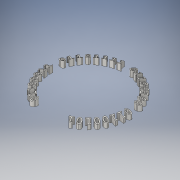
# Autodesk Inventor part: Team Pin Code-numbers
Saved by Autodesk Inventor 2016 (Build 200138000, 138)
## iProperties
Created: 2016-02-20
Part Number: Team Pin Code-numbers
Material: Generic
Document SubType Name: Modeling
Designer: RoksBot
Density: 1 g/cm^3
Appearance: White
Author: RoksBot
Autodesk Inventor part; units mm, degrees
ref_plane "YZ Plane" through (0, 0, 0) normal (1, 0, 0) x (0, 1, 0)
ref_plane "XZ Plane" through (0, 0, 0) normal (0, 1, 0) x (-1, 0, 0)
ref_plane "XY Plane" through (0, 0, 0) normal (0, 0, 1) x (1, 0, 0)
sketch "Sketch1" plane through (0, 0, 0) normal (0, 0, 1) x (1, 0, 0)
  line L0 (0, 0) -> (0, 8.6646) construction
  line L1 (20.9931, 1.27) -> (20.9931, 5.715)
  line L2 (20.9931, 5.715) -> (27.9781, 3.81)
  line L3 (27.9781, 3.81) -> (27.9781, 0)
  line L4 (27.9781, 0) -> (20.9931, 0)
  line L5 (20.9931, 1.27) -> (18.4531, 1.27)
  line L6 (18.4531, 1.27) -> (18.4531, 0)
  line L7 (18.4531, 0) -> (20.9931, 0)
  dimension "d0" = 20.9931
  dimension "d1" = 4.445
  dimension "d2" = 1.27
  dimension "d3" = 2.54
  dimension "d4" = 3.81
  dimension "d5" = 6.985
  constraints: 16 end point, 2 parallel, 2 perpendicular, 2 vertical, 1 horizontal, 1 horizontal alignment
  measures "d0" distance between parallel lines of L0 L1
  measures "d1" distance from line of L5 L1.end
  measures "d2" distance of L5.end L6.end
  measures "d3" distance between parallel lines of L1 L6
  measures "d4" distance of L2.end L3.end
  measures "d5" distance between parallel lines of L1 L3
revolve "Revolution1" add sketch "Sketch1" angle 360 about axis through (0, 0, 0) along (0, 1, 0)
sketch "Sketch2" plane through (0, 1.27, 0) normal (0, 1, 0) x (1, 0, 0)
  circle A0 centre (0, 0) radius 18.4531 projected
  circle A1 centre (0, 0) radius 27.9781 projected
  circle A2 centre (0, 0) radius 20.9931 projected
  circle A3 centre (0, 0) radius 22.8981
  line L0 (-12.5777, -21.7947) -> (-12.2792, -21.2089)
  spline S0 degree 2 poles (-12.2792, -21.2089) (-12.0125, -20.6853) (-10.9221, -20.0372) (-10.36, -20.3236) knots 0 0 0 1 2 2 2
  spline S1 degree 2 poles (-10.36, -20.3236) (-10.0346, -20.4894) (-9.7325, -21.001) (-9.7235, -21.9707) (-9.9421, -22.3997) knots 0 0 0 1 2 3 3 3
  line L1 (-9.9421, -22.3997) -> (-10.2405, -22.9854)
  spline S2 degree 2 poles (-10.2405, -22.9854) (-10.5058, -23.5061) (-11.5947, -24.1587) (-12.1568, -23.8723) knots 0 0 0 1 2 2 2
  spline S3 degree 2 poles (-12.1568, -23.8723) (-12.4793, -23.708) (-12.7828, -23.1994) (-12.7977, -22.2266) (-12.5777, -21.7947) knots 0 0 0 1 2 3 3 3
  spline S4 degree 2 poles (-12.0422, -22.0675) (-12.2653, -22.5054) (-12.1885, -22.9544) knots 0 0 0 1 1 1
  spline S5 degree 2 poles (-12.1885, -22.9544) (-12.1414, -23.2057) (-11.8899, -23.3338) knots 0 0 0 1 1 1
  spline S6 degree 2 poles (-11.8899, -23.3338) (-11.6444, -23.4589) (-11.3895, -23.3391) knots 0 0 0 1 1 1
  spline S7 degree 2 poles (-11.3895, -23.3391) (-11.0021, -23.1564) (-10.776, -22.7126) knots 0 0 0 1 1 1
  line L2 (-10.776, -22.7126) -> (-10.4776, -22.1268)
  spline S8 degree 2 poles (-10.4776, -22.1268) (-10.253, -21.686) (-10.3342, -21.2385) knots 0 0 0 1 1 1
  spline S9 degree 2 poles (-10.3342, -21.2385) (-10.3784, -20.9887) (-10.6328, -20.859) knots 0 0 0 1 1 1
  spline S10 degree 2 poles (-10.6328, -20.859) (-10.8754, -20.7355) (-11.1302, -20.8553) knots 0 0 0 1 1 1
  spline S11 degree 2 poles (-11.1302, -20.8553) (-11.5177, -21.038) (-11.7438, -21.4817) knots 0 0 0 1 1 1
  line L3 (-11.7438, -21.4817) -> (-12.0422, -22.0675)
  line L4 (-15.9925, -21.4944) -> (-14.0587, -18.8322)
  line L5 (-14.0587, -18.8322) -> (-14.5503, -18.4751)
  spline S12 degree 2 poles (-14.5503, -18.4751) (-14.733, -18.3425) (-14.7859, -18.0989) (-14.7059, -17.9887) knots 0 0 0 1 2 2 2
  spline S13 degree 2 poles (-14.7059, -17.9887) (-14.6259, -17.8786) (-14.3798, -17.8562) (-14.1971, -17.9889) knots 0 0 0 1 2 2 2
  line L6 (-14.1971, -17.9889) -> (-12.7277, -19.0563)
  spline S14 degree 2 poles (-12.7277, -19.0563) (-12.545, -19.189) (-12.4922, -19.4325) (-12.5722, -19.5427) knots 0 0 0 1 2 2 2
  spline S15 degree 2 poles (-12.5722, -19.5427) (-12.6522, -19.6528) (-12.8982, -19.6752) (-13.0809, -19.5425) knots 0 0 0 1 2 2 2
  line L7 (-13.0809, -19.5425) -> (-13.5725, -19.1854)
  line L8 (-13.5725, -19.1854) -> (-15.0457, -21.2136)
  line L9 (-15.0457, -21.2136) -> (-14.5286, -21.4169)
  spline S16 degree 2 poles (-14.5286, -21.4169) (-14.4023, -21.4635) (-14.3513, -21.5005) knots 0 0 0 1 1 1
  spline S17 degree 2 poles (-14.3513, -21.5005) (-14.2573, -21.5688) (-14.2303, -21.8141) (-14.3083, -21.9216) knots 0 0 0 1 2 2 2
  spline S18 degree 2 poles (-14.3083, -21.9216) (-14.3786, -22.0183) (-14.558, -22.0562) (-14.7477, -21.9841) knots 0 0 0 1 2 2 2
  line L10 (-14.7477, -21.9841) -> (-15.9925, -21.4944)
  line L11 (-19.1566, -18.7295) -> (-16.8304, -16.4024)
  line L12 (-16.8304, -16.4024) -> (-17.2601, -15.9728)
  spline S19 degree 2 poles (-17.2601, -15.9728) (-17.4198, -15.8132) (-17.4339, -15.5643) (-17.3377, -15.4681) knots 0 0 0 1 2 2 2
  spline S20 degree 2 poles (-17.3377, -15.4681) (-17.2415, -15.3718) (-16.9949, -15.3882) (-16.8353, -15.5478) knots 0 0 0 1 2 2 2
  line L13 (-16.8353, -15.5478) -> (-15.5508, -16.8318)
  spline S21 degree 2 poles (-15.5508, -16.8318) (-15.3911, -16.9914) (-15.377, -17.2403) (-15.4732, -17.3365) knots 0 0 0 1 2 2 2
  spline S22 degree 2 poles (-15.4732, -17.3365) (-15.5694, -17.4328) (-15.816, -17.4164) (-15.9756, -17.2568) knots 0 0 0 1 2 2 2
  line L14 (-15.9756, -17.2568) -> (-16.4054, -16.8273)
  line L15 (-16.4054, -16.8273) -> (-18.1776, -18.6002)
  line L16 (-18.1776, -18.6002) -> (-17.6986, -18.8818)
  spline S23 degree 2 poles (-17.6986, -18.8818) (-17.5812, -18.9475) (-17.5366, -18.9921) knots 0 0 0 1 1 1
  spline S24 degree 2 poles (-17.5366, -18.9921) (-17.4544, -19.0743) (-17.4661, -19.3208) (-17.56, -19.4147) knots 0 0 0 1 2 2 2
  spline S25 degree 2 poles (-17.56, -19.4147) (-17.6445, -19.4993) (-17.8276, -19.5087) (-18.0037, -19.4078) knots 0 0 0 1 2 2 2
  line L17 (-18.0037, -19.4078) -> (-19.1566, -18.7295)
  line L18 (-21.0982, -13.7139) -> (-20.5665, -13.3273)
  spline S26 degree 2 poles (-20.5665, -13.3273) (-20.0911, -12.9818) (-18.8254, -12.899) (-18.4545, -13.4093) knots 0 0 0 1 2 2 2
  spline S27 degree 2 poles (-18.4545, -13.4093) (-18.2397, -13.7047) (-18.2027, -14.2977) (-18.6347, -15.1659) (-19.0242, -15.449) knots 0 0 0 1 2 3 3 3
  line L19 (-19.0242, -15.449) -> (-19.5559, -15.8355)
  spline S28 degree 2 poles (-19.5559, -15.8355) (-20.0286, -16.1792) (-21.295, -16.2665) (-21.666, -15.7562) knots 0 0 0 1 2 2 2
  spline S29 degree 2 poles (-21.666, -15.7562) (-21.8788, -15.4635) (-21.9185, -14.8725) (-21.4903, -13.9989) (-21.0982, -13.7139) knots 0 0 0 1 2 3 3 3
  spline S30 degree 2 poles (-20.7449, -14.2) (-21.1423, -14.4889) (-21.2777, -14.9239) knots 0 0 0 1 1 1
  spline S31 degree 2 poles (-21.2777, -14.9239) (-21.3497, -15.1692) (-21.1838, -15.3975) knots 0 0 0 1 1 1
  spline S32 degree 2 poles (-21.1838, -15.3975) (-21.0218, -15.6204) (-20.7403, -15.6293) knots 0 0 0 1 1 1
  spline S33 degree 2 poles (-20.7403, -15.6293) (-20.3121, -15.6423) (-19.9093, -15.3494) knots 0 0 0 1 1 1
  line L20 (-19.9093, -15.3494) -> (-19.3775, -14.9629)
  spline S34 degree 2 poles (-19.3775, -14.9629) (-18.9774, -14.672) (-18.8467, -14.2363) knots 0 0 0 1 1 1
  spline S35 degree 2 poles (-18.8467, -14.2363) (-18.7727, -13.9936) (-18.9406, -13.7627) knots 0 0 0 1 1 1
  spline S36 degree 2 poles (-18.9406, -13.7627) (-19.1007, -13.5425) (-19.3821, -13.5336) knots 0 0 0 1 1 1
  spline S37 degree 2 poles (-19.3821, -13.5336) (-19.8103, -13.5206) (-20.2131, -13.8134) knots 0 0 0 1 1 1
  line L21 (-20.2131, -13.8134) -> (-20.7449, -14.2)
  line L22 (-22.983, -10.2463) -> (-22.3974, -9.9477)
  spline S38 degree 2 poles (-22.3974, -9.9477) (-21.8738, -9.6807) (-20.6107, -9.7969) (-20.3241, -10.3589) knots 0 0 0 1 2 2 2
  spline S39 degree 2 poles (-20.3241, -10.3589) (-20.1582, -10.6842) (-20.2144, -11.2757) (-20.7769, -12.0656) (-21.2058, -12.2844) knots 0 0 0 1 2 3 3 3
  line L23 (-21.2058, -12.2844) -> (-21.7914, -12.583)
  spline S40 degree 2 poles (-21.7914, -12.583) (-22.312, -12.8485) (-23.5765, -12.7368) (-23.8631, -12.1748) knots 0 0 0 1 2 2 2
  spline S41 degree 2 poles (-23.8631, -12.1748) (-24.0276, -11.8524) (-23.9743, -11.2624) (-23.4149, -10.4665) (-22.983, -10.2463) knots 0 0 0 1 2 3 3 3
  spline S42 degree 2 poles (-22.71, -10.7817) (-23.1478, -11.0049) (-23.3495, -11.4134) knots 0 0 0 1 1 1
  spline S43 degree 2 poles (-23.3495, -11.4134) (-23.459, -11.6444) (-23.3308, -11.8958) knots 0 0 0 1 1 1
  spline S44 degree 2 poles (-23.3308, -11.8958) (-23.2056, -12.1413) (-22.929, -12.1941) knots 0 0 0 1 1 1
  spline S45 degree 2 poles (-22.929, -12.1941) (-22.5081, -12.2739) (-22.0644, -12.0476) knots 0 0 0 1 1 1
  line L24 (-22.0644, -12.0476) -> (-21.4788, -11.749)
  spline S46 degree 2 poles (-21.4788, -11.749) (-21.0381, -11.5242) (-20.8408, -11.1143) knots 0 0 0 1 1 1
  spline S47 degree 2 poles (-20.8408, -11.1143) (-20.7298, -10.8863) (-20.8595, -10.6319) knots 0 0 0 1 1 1
  spline S48 degree 2 poles (-20.8595, -10.6319) (-20.9832, -10.3893) (-21.2598, -10.3366) knots 0 0 0 1 1 1
  spline S49 degree 2 poles (-21.2598, -10.3366) (-21.6807, -10.2568) (-22.1244, -10.483) knots 0 0 0 1 1 1
  line L25 (-22.1244, -10.483) -> (-22.71, -10.7817)
  line L26 (-24.3025, -6.5267) -> (-23.6773, -6.3233)
  spline S50 degree 2 poles (-23.6773, -6.3233) (-23.1185, -6.1414) (-21.8891, -6.4537) (-21.6939, -7.0536) knots 0 0 0 1 2 2 2
  spline S51 degree 2 poles (-21.6939, -7.0536) (-21.5809, -7.4009) (-21.7288, -7.9763) (-22.4079, -8.6686) (-22.8657, -8.8176) knots 0 0 0 1 2 3 3 3
  line L27 (-22.8657, -8.8176) -> (-23.4909, -9.021)
  spline S52 degree 2 poles (-23.4909, -9.021) (-24.0465, -9.2018) (-25.2781, -8.8937) (-25.4733, -8.2938) knots 0 0 0 1 2 2 2
  spline S53 degree 2 poles (-25.4733, -8.2938) (-25.5852, -7.9497) (-25.4404, -7.3753) (-24.7634, -6.6767) (-24.3025, -6.5267) knots 0 0 0 1 2 3 3 3
  spline S54 degree 2 poles (-24.1165, -7.0982) (-24.5838, -7.2502) (-24.8469, -7.6221) knots 0 0 0 1 1 1
  spline S55 degree 2 poles (-24.8469, -7.6221) (-24.9912, -7.8332) (-24.9038, -8.1015) knots 0 0 0 1 1 1
  spline S56 degree 2 poles (-24.9038, -8.1015) (-24.8186, -8.3636) (-24.5536, -8.459) knots 0 0 0 1 1 1
  spline S57 degree 2 poles (-24.5536, -8.459) (-24.1504, -8.6036) (-23.6768, -8.4495) knots 0 0 0 1 1 1
  line L28 (-23.6768, -8.4495) -> (-23.0517, -8.2461)
  spline S58 degree 2 poles (-23.0517, -8.2461) (-22.5812, -8.093) (-22.3223, -7.719) knots 0 0 0 1 1 1
  spline S59 degree 2 poles (-22.3223, -7.719) (-22.177, -7.5111) (-22.2653, -7.2395) knots 0 0 0 1 1 1
  spline S60 degree 2 poles (-22.2653, -7.2395) (-22.3496, -6.9806) (-22.6146, -6.8853) knots 0 0 0 1 1 1
  spline S61 degree 2 poles (-22.6146, -6.8853) (-23.0178, -6.7406) (-23.4914, -6.8947) knots 0 0 0 1 1 1
  line L29 (-23.4914, -6.8947) -> (-24.1165, -7.0982)
  line L30 (-26.5057, -3.9006) -> (-23.2561, -3.3842)
  line L31 (-23.2561, -3.3842) -> (-23.3515, -2.7842)
  spline S62 degree 2 poles (-23.3515, -2.7842) (-23.3869, -2.5612) (-23.2521, -2.3515) (-23.1177, -2.3301) knots 0 0 0 1 2 2 2
  spline S63 degree 2 poles (-23.1177, -2.3301) (-22.9832, -2.3088) (-22.7934, -2.4669) (-22.758, -2.6899) knots 0 0 0 1 2 2 2
  line L32 (-22.758, -2.6899) -> (-22.473, -4.4835)
  spline S64 degree 2 poles (-22.473, -4.4835) (-22.4375, -4.7065) (-22.5723, -4.9162) (-22.7067, -4.9376) knots 0 0 0 1 2 2 2
  spline S65 degree 2 poles (-22.7067, -4.9376) (-22.8412, -4.9589) (-23.031, -4.8008) (-23.0665, -4.5778) knots 0 0 0 1 2 2 2
  line L33 (-23.0665, -4.5778) -> (-23.1618, -3.9778)
  line L34 (-23.1618, -3.9778) -> (-25.6376, -4.3711)
  line L35 (-25.6376, -4.3711) -> (-25.4154, -4.8805)
  spline S66 degree 2 poles (-25.4154, -4.8805) (-25.359, -5.0026) (-25.3491, -5.0649) knots 0 0 0 1 1 1
  spline S67 degree 2 poles (-25.3491, -5.0649) (-25.3309, -5.1797) (-25.4852, -5.3723) (-25.6164, -5.3932) knots 0 0 0 1 2 2 2
  spline S68 degree 2 poles (-25.6164, -5.3932) (-25.7344, -5.4119) (-25.8881, -5.3119) (-25.9713, -5.1268) knots 0 0 0 1 2 2 2
  line L36 (-25.9713, -5.1268) -> (-26.5057, -3.9006)
  line L37 (-26.7896, 0.2918) -> (-23.4992, 0.2937)
  line L38 (-23.4992, 0.2937) -> (-23.4996, 0.9013)
  spline S69 degree 2 poles (-23.4996, 0.9013) (-23.4997, 1.1271) (-23.3338, 1.3131) (-23.1977, 1.3132) knots 0 0 0 1 2 2 2
  spline S70 degree 2 poles (-23.1977, 1.3132) (-23.0615, 1.3133) (-22.8987, 1.1274) (-22.8986, 0.9016) knots 0 0 0 1 2 2 2
  line L39 (-22.8986, 0.9016) -> (-22.8976, -0.9145)
  spline S71 degree 2 poles (-22.8976, -0.9145) (-22.8975, -1.1403) (-23.0634, -1.3263) (-23.1995, -1.3264) knots 0 0 0 1 2 2 2
  spline S72 degree 2 poles (-23.1995, -1.3264) (-23.3356, -1.3265) (-23.4984, -1.1407) (-23.4985, -0.9149) knots 0 0 0 1 2 2 2
  line L40 (-23.4985, -0.9149) -> (-23.4989, -0.3073)
  line L41 (-23.4989, -0.3073) -> (-26.0057, -0.3087)
  line L42 (-26.0057, -0.3087) -> (-25.8659, -0.8465)
  spline S73 degree 2 poles (-25.8659, -0.8465) (-25.8293, -0.976) (-25.8293, -1.0391) knots 0 0 0 1 1 1
  spline S74 degree 2 poles (-25.8293, -1.0391) (-25.8292, -1.1553) (-26.0118, -1.3214) (-26.1446, -1.3215) knots 0 0 0 1 2 2 2
  spline S75 degree 2 poles (-26.1446, -1.3215) (-26.2641, -1.3215) (-26.4003, -1.1988) (-26.4535, -1.0029) knots 0 0 0 1 2 2 2
  line L43 (-26.4535, -1.0029) -> (-26.7896, 0.2918)
  line L44 (-23.5001, 8.9973) -> (-22.8747, 8.7946)
  spline S76 degree 2 poles (-22.8747, 8.7946) (-22.3157, 8.6134) (-21.5043, 7.6384) (-21.6988, 7.0383) knots 0 0 0 1 2 2 2
  spline S77 degree 2 poles (-21.6988, 7.0383) (-21.8115, 6.6908) (-22.2693, 6.3122) (-23.2255, 6.1509) (-23.6835, 6.2994) knots 0 0 0 1 2 3 3 3
  line L45 (-23.6835, 6.2994) -> (-24.3089, 6.5021)
  spline S78 degree 2 poles (-24.3089, 6.5021) (-24.8648, 6.6822) (-25.6803, 7.6551) (-25.4858, 8.2552) knots 0 0 0 1 2 2 2
  spline S79 degree 2 poles (-25.4858, 8.2552) (-25.3742, 8.5995) (-24.9196, 8.9792) (-23.9613, 9.1467) (-23.5001, 8.9973) knots 0 0 0 1 2 3 3 3
  spline S80 degree 2 poles (-23.6854, 8.4256) (-24.1529, 8.5771) (-24.5843, 8.4307) knots 0 0 0 1 1 1
  spline S81 degree 2 poles (-24.5843, 8.4307) (-24.825, 8.3447) (-24.9121, 8.0762) knots 0 0 0 1 1 1
  spline S82 degree 2 poles (-24.9121, 8.0762) (-24.997, 7.8141) (-24.8386, 7.5812) knots 0 0 0 1 1 1
  spline S83 degree 2 poles (-24.8386, 7.5812) (-24.5974, 7.2273) (-24.1236, 7.0737) knots 0 0 0 1 1 1
  line L46 (-24.1236, 7.0737) -> (-23.4982, 6.871)
  spline S84 degree 2 poles (-23.4982, 6.871) (-23.0276, 6.7185) (-22.5983, 6.8691) knots 0 0 0 1 1 1
  spline S85 degree 2 poles (-22.5983, 6.8691) (-22.3586, 6.9519) (-22.2705, 7.2236) knots 0 0 0 1 1 1
  spline S86 degree 2 poles (-22.2705, 7.2236) (-22.1866, 7.4825) (-22.345, 7.7154) knots 0 0 0 1 1 1
  spline S87 degree 2 poles (-22.345, 7.7154) (-22.5863, 8.0693) (-23.06, 8.2229) knots 0 0 0 1 1 1
  line L47 (-23.06, 8.2229) -> (-23.6854, 8.4256)
  line L48 (-23.7401, 12.4168) -> (-20.8071, 10.9254)
  line L49 (-20.8071, 10.9254) -> (-20.5317, 11.467)
  spline S88 degree 2 poles (-20.5317, 11.467) (-20.4294, 11.6682) (-20.1971, 11.7587) (-20.0758, 11.697) knots 0 0 0 1 2 2 2
  spline S89 degree 2 poles (-20.0758, 11.697) (-19.9544, 11.6353) (-19.8937, 11.3958) (-19.996, 11.1946) knots 0 0 0 1 2 2 2
  line L50 (-19.996, 11.1946) -> (-20.8193, 9.5757)
  spline S90 degree 2 poles (-20.8193, 9.5757) (-20.9216, 9.3744) (-21.1539, 9.2839) (-21.2752, 9.3456) knots 0 0 0 1 2 2 2
  spline S91 degree 2 poles (-21.2752, 9.3456) (-21.3966, 9.4073) (-21.4573, 9.6468) (-21.355, 9.8481) knots 0 0 0 1 2 2 2
  line L51 (-21.355, 9.8481) -> (-21.0795, 10.3897)
  line L52 (-21.0795, 10.3897) -> (-23.314, 11.526)
  line L53 (-23.314, 11.526) -> (-23.4335, 10.9833)
  spline S92 degree 2 poles (-23.4335, 10.9833) (-23.4597, 10.8513) (-23.4883, 10.7951) knots 0 0 0 1 1 1
  spline S93 degree 2 poles (-23.4883, 10.7951) (-23.5409, 10.6915) (-23.779, 10.6263) (-23.8974, 10.6865) knots 0 0 0 1 2 2 2
  spline S94 degree 2 poles (-23.8974, 10.6865) (-24.0039, 10.7407) (-24.0696, 10.9119) (-24.0281, 11.1106) knots 0 0 0 1 2 2 2
  line L54 (-24.0281, 11.1106) -> (-23.7401, 12.4168)
  line L55 (-21.5066, 15.9761) -> (-18.8429, 14.0444)
  line L56 (-18.8429, 14.0444) -> (-18.4862, 14.5362)
  spline S95 degree 2 poles (-18.4862, 14.5362) (-18.3537, 14.719) (-18.1101, 14.7721) (-17.9999, 14.6922) knots 0 0 0 1 2 2 2
  spline S96 degree 2 poles (-17.9999, 14.6922) (-17.8897, 14.6122) (-17.8672, 14.3662) (-17.9997, 14.1834) knots 0 0 0 1 2 2 2
  line L57 (-17.9997, 14.1834) -> (-19.066, 12.7132)
  spline S97 degree 2 poles (-19.066, 12.7132) (-19.1985, 12.5304) (-19.4421, 12.4773) (-19.5523, 12.5573) knots 0 0 0 1 2 2 2
  spline S98 degree 2 poles (-19.5523, 12.5573) (-19.6625, 12.6372) (-19.685, 12.8832) (-19.5525, 13.066) knots 0 0 0 1 2 2 2
  line L58 (-19.5525, 13.066) -> (-19.1957, 13.5579)
  line L59 (-19.1957, 13.5579) -> (-21.2251, 15.0295)
  line L60 (-21.2251, 15.0295) -> (-21.428, 14.5122)
  spline S99 degree 2 poles (-21.428, 14.5122) (-21.4744, 14.386) (-21.5115, 14.3349) knots 0 0 0 1 1 1
  spline S100 degree 2 poles (-21.5115, 14.3349) (-21.5797, 14.2408) (-21.825, 14.2136) (-21.9325, 14.2916) knots 0 0 0 1 2 2 2
  spline S101 degree 2 poles (-21.9325, 14.2916) (-22.0293, 14.3618) (-22.0673, 14.5412) (-21.9953, 14.7309) knots 0 0 0 1 2 2 2
  line L61 (-21.9953, 14.7309) -> (-21.5066, 15.9761)
  line L62 (-16.8584, 18.6816) -> (-16.3931, 18.2172)
  spline S102 degree 2 poles (-16.3931, 18.2172) (-15.9771, 17.802) (-15.6965, 16.565) (-16.1422, 16.1185) knots 0 0 0 1 2 2 2
  spline S103 degree 2 poles (-16.1422, 16.1185) (-16.4002, 15.86) (-16.98, 15.7303) (-17.9053, 16.0206) (-18.246, 16.3607) knots 0 0 0 1 2 3 3 3
  line L63 (-18.246, 16.3607) -> (-18.7113, 16.8251)
  spline S104 degree 2 poles (-18.7113, 16.8251) (-19.1249, 17.2379) (-19.4102, 18.4749) (-18.9646, 18.9214) knots 0 0 0 1 2 2 2
  spline S105 degree 2 poles (-18.9646, 18.9214) (-18.7089, 19.1776) (-18.1315, 19.3096) (-17.2015, 19.0241) (-16.8584, 18.6816) knots 0 0 0 1 2 3 3 3
  spline S106 degree 2 poles (-17.2829, 18.2563) (-17.6307, 18.6034) (-18.0815, 18.6687) knots 0 0 0 1 1 1
  spline S107 degree 2 poles (-18.0815, 18.6687) (-18.3351, 18.7013) (-18.5345, 18.5016) knots 0 0 0 1 1 1
  spline S108 degree 2 poles (-18.5345, 18.5016) (-18.7292, 18.3065) (-18.6937, 18.0272) knots 0 0 0 1 1 1
  spline S109 degree 2 poles (-18.6937, 18.0272) (-18.6393, 17.6023) (-18.2868, 17.2504) knots 0 0 0 1 1 1
  line L64 (-18.2868, 17.2504) -> (-17.8215, 16.786)
  spline S110 degree 2 poles (-17.8215, 16.786) (-17.4713, 16.4365) (-17.0205, 16.3759) knots 0 0 0 1 1 1
  spline S111 degree 2 poles (-17.0205, 16.3759) (-16.7693, 16.341) (-16.5675, 16.5431) knots 0 0 0 1 1 1
  spline S112 degree 2 poles (-16.5675, 16.5431) (-16.3752, 16.7358) (-16.4107, 17.0151) knots 0 0 0 1 1 1
  spline S113 degree 2 poles (-16.4107, 17.0151) (-16.4651, 17.44) (-16.8176, 17.7918) knots 0 0 0 1 1 1
  line L65 (-16.8176, 17.7918) -> (-17.2829, 18.2563)
  line L66 (-15.5204, 21.8377) -> (-13.5837, 19.1777)
  line L67 (-13.5837, 19.1777) -> (-13.0925, 19.5354)
  spline S114 degree 2 poles (-13.0925, 19.5354) (-12.91, 19.6683) (-12.6619, 19.6435) (-12.5818, 19.5334) knots 0 0 0 1 2 2 2
  spline S115 degree 2 poles (-12.5818, 19.5334) (-12.5017, 19.4234) (-12.5562, 19.1824) (-12.7387, 19.0495) knots 0 0 0 1 2 2 2
  line L68 (-12.7387, 19.0495) -> (-14.207, 17.9805)
  spline S116 degree 2 poles (-14.207, 17.9805) (-14.3895, 17.8476) (-14.6375, 17.8724) (-14.7176, 17.9824) knots 0 0 0 1 2 2 2
  spline S117 degree 2 poles (-14.7176, 17.9824) (-14.7978, 18.0925) (-14.7432, 18.3334) (-14.5607, 18.4663) knots 0 0 0 1 2 2 2
  line L69 (-14.5607, 18.4663) -> (-14.0695, 18.824)
  line L70 (-14.0695, 18.824) -> (-15.545, 20.8505)
  line L71 (-15.545, 20.8505) -> (-15.8978, 20.4212)
  spline S118 degree 2 poles (-15.8978, 20.4212) (-15.981, 20.3154) (-16.032, 20.2783) knots 0 0 0 1 1 1
  spline S119 degree 2 poles (-16.032, 20.2783) (-16.1259, 20.2099) (-16.3676, 20.2598) (-16.4458, 20.3671) knots 0 0 0 1 2 2 2
  spline S120 degree 2 poles (-16.4458, 20.3671) (-16.5161, 20.4638) (-16.497, 20.6461) (-16.3699, 20.8044) knots 0 0 0 1 2 2 2
  line L72 (-16.3699, 20.8044) -> (-15.5204, 21.8377)
  line L73 (-11.915, 23.9959) -> (-10.418, 21.0658)
  line L74 (-10.418, 21.0658) -> (-9.8769, 21.3422)
  spline S121 degree 2 poles (-9.8769, 21.3422) (-9.6759, 21.4449) (-9.4347, 21.3817) (-9.3728, 21.2605) knots 0 0 0 1 2 2 2
  spline S122 degree 2 poles (-9.3728, 21.2605) (-9.3109, 21.1392) (-9.4024, 20.9098) (-9.6035, 20.807) knots 0 0 0 1 2 2 2
  line L75 (-9.6035, 20.807) -> (-11.2208, 19.9807)
  spline S123 degree 2 poles (-11.2208, 19.9807) (-11.4219, 19.878) (-11.663, 19.9412) (-11.7249, 20.0625) knots 0 0 0 1 2 2 2
  spline S124 degree 2 poles (-11.7249, 20.0625) (-11.7868, 20.1837) (-11.6953, 20.4132) (-11.4942, 20.5159) knots 0 0 0 1 2 2 2
  line L76 (-11.4942, 20.5159) -> (-10.9531, 20.7923)
  line L77 (-10.9531, 20.7923) -> (-12.0937, 23.0246)
  line L78 (-12.0937, 23.0246) -> (-12.5092, 22.6557)
  spline S125 degree 2 poles (-12.5092, 22.6557) (-12.6079, 22.5643) (-12.6641, 22.5356) knots 0 0 0 1 1 1
  spline S126 degree 2 poles (-12.6641, 22.5356) (-12.7676, 22.4827) (-12.9985, 22.5698) (-13.0589, 22.6881) knots 0 0 0 1 2 2 2
  spline S127 degree 2 poles (-13.0589, 22.6881) (-13.1133, 22.7945) (-13.0658, 22.9716) (-12.9156, 23.1081) knots 0 0 0 1 2 2 2
  line L79 (-12.9156, 23.1081) -> (-11.915, 23.9959)
  line L80 (-8.0165, 25.5637) -> (-6.996, 22.4356)
  line L81 (-6.996, 22.4356) -> (-6.4184, 22.624)
  spline S128 degree 2 poles (-6.4184, 22.624) (-6.2037, 22.6941) (-5.9755, 22.5939) (-5.9333, 22.4645) knots 0 0 0 1 2 2 2
  spline S129 degree 2 poles (-5.9333, 22.4645) (-5.891, 22.3351) (-6.0173, 22.1227) (-6.232, 22.0527) knots 0 0 0 1 2 2 2
  line L82 (-6.232, 22.0527) -> (-7.9586, 21.4894)
  spline S130 degree 2 poles (-7.9586, 21.4894) (-8.1733, 21.4194) (-8.4015, 21.5196) (-8.4437, 21.649) knots 0 0 0 1 2 2 2
  spline S131 degree 2 poles (-8.4437, 21.649) (-8.486, 21.7784) (-8.3596, 21.9908) (-8.145, 22.0608) knots 0 0 0 1 2 2 2
  line L83 (-8.145, 22.0608) -> (-7.5674, 22.2492)
  line L84 (-7.5674, 22.2492) -> (-8.3448, 24.6324)
  line L85 (-8.3448, 24.6324) -> (-8.8129, 24.333)
  spline S132 degree 2 poles (-8.8129, 24.333) (-8.9247, 24.2581) (-8.9847, 24.2386) knots 0 0 0 1 1 1
  spline S133 degree 2 poles (-8.9847, 24.2386) (-9.0952, 24.2025) (-9.3096, 24.3246) (-9.3508, 24.4509) knots 0 0 0 1 2 2 2
  spline S134 degree 2 poles (-9.3508, 24.4509) (-9.3879, 24.5645) (-9.3133, 24.7321) (-9.1435, 24.8433) knots 0 0 0 1 2 2 2
  line L86 (-9.1435, 24.8433) -> (-8.0165, 25.5637)
  line L87 (-3.9208, 26.5028) -> (-3.402, 23.2535)
  line L88 (-3.402, 23.2535) -> (-2.802, 23.3493)
  spline S135 degree 2 poles (-2.802, 23.3493) (-2.579, 23.3849) (-2.3692, 23.2503) (-2.3477, 23.1159) knots 0 0 0 1 2 2 2
  spline S136 degree 2 poles (-2.3477, 23.1159) (-2.3263, 22.9815) (-2.4842, 22.7915) (-2.7072, 22.7559) knots 0 0 0 1 2 2 2
  line L89 (-2.7072, 22.7559) -> (-4.5007, 22.4695)
  spline S137 degree 2 poles (-4.5007, 22.4695) (-4.7236, 22.4339) (-4.9334, 22.5685) (-4.9549, 22.703) knots 0 0 0 1 2 2 2
  spline S138 degree 2 poles (-4.9549, 22.703) (-4.9763, 22.8374) (-4.8184, 23.0274) (-4.5954, 23.063) knots 0 0 0 1 2 2 2
  line L90 (-4.5954, 23.063) -> (-3.9954, 23.1588)
  line L91 (-3.9954, 23.1588) -> (-4.3907, 25.6342)
  line L92 (-4.3907, 25.6342) -> (-4.8998, 25.4117)
  spline S139 degree 2 poles (-4.8998, 25.4117) (-5.0219, 25.3552) (-5.0842, 25.3453) knots 0 0 0 1 1 1
  spline S140 degree 2 poles (-5.0842, 25.3453) (-5.199, 25.327) (-5.3917, 25.4811) (-5.4127, 25.6123) knots 0 0 0 1 2 2 2
  spline S141 degree 2 poles (-5.4127, 25.6123) (-5.4315, 25.7303) (-5.3317, 25.8841) (-5.1466, 25.9674) knots 0 0 0 1 2 2 2
  line L93 (-5.1466, 25.9674) -> (-3.9208, 26.5028)
  line L94 (5.1934, 24.6219) -> (5.0915, 23.9724)
  spline S142 degree 2 poles (5.0915, 23.9724) (5.0003, 23.3918) (4.1649, 22.4373) (3.5417, 22.5352) knots 0 0 0 1 2 2 2
  spline S143 degree 2 poles (3.5417, 22.5352) (3.1809, 22.5918) (2.735, 22.9844) (2.4255, 23.9035) (2.5002, 24.3791) knots 0 0 0 1 2 3 3 3
  line L95 (2.5002, 24.3791) -> (2.6021, 25.0285)
  spline S144 degree 2 poles (2.6021, 25.0285) (2.6927, 25.6058) (3.5253, 26.5641) (4.1486, 26.4663) knots 0 0 0 1 2 2 2
  spline S145 degree 2 poles (4.1486, 26.4663) (4.5061, 26.4102) (4.9525, 26.0208) (5.2685, 25.1007) (5.1934, 24.6219) knots 0 0 0 1 2 3 3 3
  spline S146 degree 2 poles (4.5997, 24.715) (4.6759, 25.2005) (4.4635, 25.6035) knots 0 0 0 1 1 1
  spline S147 degree 2 poles (4.4635, 25.6035) (4.3408, 25.8278) (4.062, 25.8715) knots 0 0 0 1 1 1
  spline S148 degree 2 poles (4.062, 25.8715) (3.7897, 25.9143) (3.5847, 25.7213) knots 0 0 0 1 1 1
  spline S149 degree 2 poles (3.5847, 25.7213) (3.273, 25.4274) (3.1958, 24.9354) knots 0 0 0 1 1 1
  line L96 (3.1958, 24.9354) -> (3.0939, 24.2859)
  spline S150 degree 2 poles (3.0939, 24.2859) (3.0172, 23.7972) (3.2333, 23.3969) knots 0 0 0 1 1 1
  spline S151 degree 2 poles (3.2333, 23.3969) (3.3528, 23.1731) (3.6349, 23.1289) knots 0 0 0 1 1 1
  spline S152 degree 2 poles (3.6349, 23.1289) (3.9038, 23.0866) (4.1089, 23.2796) knots 0 0 0 1 1 1
  spline S153 degree 2 poles (4.1089, 23.2796) (4.4205, 23.5735) (4.4978, 24.0656) knots 0 0 0 1 1 1
  line L97 (4.4978, 24.0656) -> (4.5997, 24.715)
  line L98 (8.5328, 25.3961) -> (7.5206, 22.2652)
  line L99 (7.5206, 22.2652) -> (8.0988, 22.0783)
  spline S154 degree 2 poles (8.0988, 22.0783) (8.3136, 22.0089) (8.4395, 21.7937) (8.3976, 21.6642) knots 0 0 0 1 2 2 2
  spline S155 degree 2 poles (8.3976, 21.6642) (8.3557, 21.5347) (8.1287, 21.4371) (7.9139, 21.5065) knots 0 0 0 1 2 2 2
  line L100 (7.9139, 21.5065) -> (6.1858, 22.0652)
  spline S156 degree 2 poles (6.1858, 22.0652) (5.971, 22.1346) (5.8451, 22.3498) (5.887, 22.4793) knots 0 0 0 1 2 2 2
  spline S157 degree 2 poles (5.887, 22.4793) (5.9289, 22.6088) (6.1558, 22.7064) (6.3707, 22.637) knots 0 0 0 1 2 2 2
  line L101 (6.3707, 22.637) -> (6.9488, 22.4501)
  line L102 (6.9488, 22.4501) -> (7.7199, 24.8353)
  line L103 (7.7199, 24.8353) -> (7.1652, 24.8681)
  spline S158 degree 2 poles (7.1652, 24.8681) (7.0308, 24.8732) (6.9707, 24.8926) knots 0 0 0 1 1 1
  spline S159 degree 2 poles (6.9707, 24.8926) (6.8602, 24.9283) (6.7584, 25.1532) (6.7992, 25.2795) knots 0 0 0 1 2 2 2
  spline S160 degree 2 poles (6.7992, 25.2795) (6.836, 25.3933) (6.9948, 25.485) (7.1975, 25.4753) knots 0 0 0 1 2 2 2
  line L104 (7.1975, 25.4753) -> (8.5328, 25.3961)
  line L105 (12.3987, 23.7495) -> (10.9095, 20.8155)
  line L106 (10.9095, 20.8155) -> (11.4513, 20.5405)
  spline S161 degree 2 poles (11.4513, 20.5405) (11.6526, 20.4383) (11.7433, 20.2061) (11.6817, 20.0847) knots 0 0 0 1 2 2 2
  spline S162 degree 2 poles (11.6817, 20.0847) (11.6201, 19.9633) (11.3806, 19.9024) (11.1793, 20.0046) knots 0 0 0 1 2 2 2
  line L107 (11.1793, 20.0046) -> (9.5598, 20.8266)
  spline S163 degree 2 poles (9.5598, 20.8266) (9.3585, 20.9288) (9.2678, 21.1609) (9.3294, 21.2823) knots 0 0 0 1 2 2 2
  spline S164 degree 2 poles (9.3294, 21.2823) (9.391, 21.4037) (9.6305, 21.4646) (9.8318, 21.3625) knots 0 0 0 1 2 2 2
  line L108 (9.8318, 21.3625) -> (10.3736, 21.0875)
  line L109 (10.3736, 21.0875) -> (11.5082, 23.3228)
  line L110 (11.5082, 23.3228) -> (10.9654, 23.4419)
  spline S165 degree 2 poles (10.9654, 23.4419) (10.8334, 23.4679) (10.7772, 23.4965) knots 0 0 0 1 1 1
  spline S166 degree 2 poles (10.7772, 23.4965) (10.6736, 23.5491) (10.6082, 23.7871) (10.6683, 23.9055) knots 0 0 0 1 2 2 2
  spline S167 degree 2 poles (10.6683, 23.9055) (10.7224, 24.0121) (10.8935, 24.0779) (11.0923, 24.0366) knots 0 0 0 1 2 2 2
  line L111 (11.0923, 24.0366) -> (12.3987, 23.7495)
  line L112 (15.801, 19.5841) -> (15.4154, 19.0516)
  spline S168 degree 2 poles (15.4154, 19.0516) (15.0708, 18.5756) (13.8932, 18.1042) (13.3822, 18.4741) knots 0 0 0 1 2 2 2
  spline S169 degree 2 poles (13.3822, 18.4741) (13.0864, 18.6883) (12.8672, 19.2405) (13.0085, 20.1999) (13.2908, 20.5899) knots 0 0 0 1 2 3 3 3
  line L113 (13.2908, 20.5899) -> (13.6764, 21.1224)
  spline S170 degree 2 poles (13.6764, 21.1224) (14.0191, 21.5957) (15.1959, 22.0718) (15.7069, 21.7018) knots 0 0 0 1 2 2 2
  spline S171 degree 2 poles (15.7069, 21.7018) (16, 21.4896) (16.2211, 20.94) (16.0852, 19.9767) (15.801, 19.5841) knots 0 0 0 1 2 3 3 3
  spline S172 degree 2 poles (15.3142, 19.9365) (15.6024, 20.3346) (15.596, 20.7901) knots 0 0 0 1 1 1
  spline S173 degree 2 poles (15.596, 20.7901) (15.5884, 21.0456) (15.3598, 21.2111) knots 0 0 0 1 1 1
  spline S174 degree 2 poles (15.3598, 21.2111) (15.1366, 21.3728) (14.8663, 21.2938) knots 0 0 0 1 1 1
  spline S175 degree 2 poles (14.8663, 21.2938) (14.4552, 21.1733) (14.1631, 20.7699) knots 0 0 0 1 1 1
  line L114 (14.1631, 20.7699) -> (13.7776, 20.2375)
  spline S176 degree 2 poles (13.7776, 20.2375) (13.4875, 19.8367) (13.4984, 19.382) knots 0 0 0 1 1 1
  spline S177 degree 2 poles (13.4984, 19.382) (13.5034, 19.1284) (13.7346, 18.9609) knots 0 0 0 1 1 1
  spline S178 degree 2 poles (13.7346, 18.9609) (13.9552, 18.8012) (14.2255, 18.8802) knots 0 0 0 1 1 1
  spline S179 degree 2 poles (14.2255, 18.8802) (14.6366, 19.0006) (14.9286, 19.404) knots 0 0 0 1 1 1
  line L115 (14.9286, 19.404) -> (15.3142, 19.9365)
  line L116 (18.6688, 16.8726) -> (18.2047, 16.4069)
  spline S180 degree 2 poles (18.2047, 16.4069) (17.7899, 15.9907) (16.5531, 15.7092) (16.1062, 16.1545) knots 0 0 0 1 2 2 2
  spline S181 degree 2 poles (16.1062, 16.1545) (15.8475, 16.4123) (15.7174, 16.992) (16.0069, 17.9175) (16.3468, 18.2585) knots 0 0 0 1 2 3 3 3
  line L117 (16.3468, 18.2585) -> (16.8108, 18.7242)
  spline S182 degree 2 poles (16.8108, 18.7242) (17.2233, 19.1381) (18.4601, 19.4243) (18.907, 18.979) knots 0 0 0 1 2 2 2
  spline S183 degree 2 poles (18.907, 18.979) (19.1633, 18.7235) (19.2958, 18.1462) (19.0109, 17.216) (18.6688, 16.8726) knots 0 0 0 1 2 3 3 3
  spline S184 degree 2 poles (18.2431, 17.2968) (18.59, 17.6449) (18.6549, 18.0958) knots 0 0 0 1 1 1
  spline S185 degree 2 poles (18.6549, 18.0958) (18.6874, 18.3494) (18.4875, 18.5486) knots 0 0 0 1 1 1
  spline S186 degree 2 poles (18.4875, 18.5486) (18.2923, 18.7431) (18.0129, 18.7074) knots 0 0 0 1 1 1
  spline S187 degree 2 poles (18.0129, 18.7074) (17.5881, 18.6527) (17.2365, 18.2999) knots 0 0 0 1 1 1
  line L118 (17.2365, 18.2999) -> (16.7724, 17.8343)
  spline S188 degree 2 poles (16.7724, 17.8343) (16.4232, 17.4839) (16.363, 17.033) knots 0 0 0 1 1 1
  spline S189 degree 2 poles (16.363, 17.033) (16.3282, 16.7817) (16.5304, 16.5802) knots 0 0 0 1 1 1
  spline S190 degree 2 poles (16.5304, 16.5802) (16.7233, 16.388) (17.0026, 16.4237) knots 0 0 0 1 1 1
  spline S191 degree 2 poles (17.0026, 16.4237) (17.4275, 16.4784) (17.779, 16.8312) knots 0 0 0 1 1 1
  line L119 (17.779, 16.8312) -> (18.2431, 17.2968)
  line L120 (21.8259, 15.5371) -> (19.1673, 13.5983)
  line L121 (19.1673, 13.5983) -> (19.5254, 13.1074)
  spline S192 degree 2 poles (19.5254, 13.1074) (19.6584, 12.9249) (19.6338, 12.6769) (19.5238, 12.5967) knots 0 0 0 1 2 2 2
  spline S193 degree 2 poles (19.5238, 12.5967) (19.4139, 12.5165) (19.1728, 12.5708) (19.0398, 12.7532) knots 0 0 0 1 2 2 2
  line L122 (19.0398, 12.7532) -> (17.9697, 14.2207)
  spline S194 degree 2 poles (17.9697, 14.2207) (17.8366, 14.4031) (17.8612, 14.6511) (17.9712, 14.7313) knots 0 0 0 1 2 2 2
  spline S195 degree 2 poles (17.9712, 14.7313) (18.0812, 14.8115) (18.3222, 14.7572) (18.4552, 14.5748) knots 0 0 0 1 2 2 2
  line L123 (18.4552, 14.5748) -> (18.8132, 14.0838)
  line L124 (18.8132, 14.0838) -> (20.8386, 15.5609)
  line L125 (20.8386, 15.5609) -> (20.409, 15.9133)
  spline S196 degree 2 poles (20.409, 15.9133) (20.3032, 15.9964) (20.266, 16.0474) knots 0 0 0 1 1 1
  spline S197 degree 2 poles (20.266, 16.0474) (20.1976, 16.1413) (20.2473, 16.383) (20.3546, 16.4613) knots 0 0 0 1 2 2 2
  spline S198 degree 2 poles (20.3546, 16.4613) (20.4512, 16.5317) (20.6336, 16.5127) (20.7919, 16.3857) knots 0 0 0 1 2 2 2
  line L126 (20.7919, 16.3857) -> (21.8259, 15.5371)
  line L127 (22.9674, 10.2813) -> (22.3822, 9.9818)
  spline S199 degree 2 poles (22.3822, 9.9818) (21.8591, 9.714) (20.5958, 9.8283) (20.3083, 10.3898) knots 0 0 0 1 2 2 2
  spline S200 degree 2 poles (20.3083, 10.3898) (20.1419, 10.7149) (20.1972, 11.3065) (20.7585, 12.0973) (21.187, 12.3167) knots 0 0 0 1 2 3 3 3
  line L128 (21.187, 12.3167) -> (21.7722, 12.6162)
  spline S201 degree 2 poles (21.7722, 12.6162) (22.2924, 12.8825) (23.5571, 12.7727) (23.8446, 12.2111) knots 0 0 0 1 2 2 2
  spline S202 degree 2 poles (23.8446, 12.2111) (24.0095, 11.889) (23.9571, 11.299) (23.3989, 10.5022) (22.9674, 10.2813) knots 0 0 0 1 2 3 3 3
  spline S203 degree 2 poles (22.6936, 10.8163) (23.131, 11.0402) (23.332, 11.449) knots 0 0 0 1 1 1
  spline S204 degree 2 poles (23.332, 11.449) (23.4412, 11.6802) (23.3126, 11.9314) knots 0 0 0 1 1 1
  spline S205 degree 2 poles (23.3126, 11.9314) (23.1871, 12.1767) (22.9104, 12.229) knots 0 0 0 1 1 1
  spline S206 degree 2 poles (22.9104, 12.229) (22.4894, 12.3082) (22.046, 12.0813) knots 0 0 0 1 1 1
  line L129 (22.046, 12.0813) -> (21.4608, 11.7817)
  spline S207 degree 2 poles (21.4608, 11.7817) (21.0205, 11.5563) (20.8239, 11.1461) knots 0 0 0 1 1 1
  spline S208 degree 2 poles (20.8239, 11.1461) (20.7132, 10.9178) (20.8433, 10.6637) knots 0 0 0 1 1 1
  spline S209 degree 2 poles (20.8433, 10.6637) (20.9674, 10.4213) (21.244, 10.369) knots 0 0 0 1 1 1
  spline S210 degree 2 poles (21.244, 10.369) (21.665, 10.2898) (22.1084, 10.5167) knots 0 0 0 1 1 1
  line L130 (22.1084, 10.5167) -> (22.6936, 10.8163)
  line L131 (24.2925, 6.5637) -> (23.6676, 6.3593)
  spline S211 degree 2 poles (23.6676, 6.3593) (23.1091, 6.1766) (21.8792, 6.487) (21.6831, 7.0866) knots 0 0 0 1 2 2 2
  spline S212 degree 2 poles (21.6831, 7.0866) (21.5696, 7.4338) (21.7167, 8.0094) (22.3947, 8.7027) (22.8522, 8.8524) knots 0 0 0 1 2 3 3 3
  line L132 (22.8522, 8.8524) -> (23.4771, 9.0568)
  spline S213 degree 2 poles (23.4771, 9.0568) (24.0325, 9.2384) (25.2645, 8.9322) (25.4606, 8.3326) knots 0 0 0 1 2 2 2
  spline S214 degree 2 poles (25.4606, 8.3326) (25.5731, 7.9886) (25.4292, 7.4141) (24.7532, 6.7144) (24.2925, 6.5637) knots 0 0 0 1 2 3 3 3
  spline S215 degree 2 poles (24.1057, 7.1349) (24.5727, 7.2877) (24.8352, 7.66) knots 0 0 0 1 1 1
  spline S216 degree 2 poles (24.8352, 7.66) (24.9792, 7.8712) (24.8915, 8.1395) knots 0 0 0 1 1 1
  spline S217 degree 2 poles (24.8915, 8.1395) (24.8058, 8.4014) (24.5407, 8.4964) knots 0 0 0 1 1 1
  spline S218 degree 2 poles (24.5407, 8.4964) (24.1373, 8.6404) (23.6639, 8.4856) knots 0 0 0 1 1 1
  line L133 (23.6639, 8.4856) -> (23.0391, 8.2812)
  spline S219 degree 2 poles (23.0391, 8.2812) (22.5689, 8.1274) (22.3105, 7.753) knots 0 0 0 1 1 1
  spline S220 degree 2 poles (22.3105, 7.753) (22.1655, 7.5448) (22.2543, 7.2735) knots 0 0 0 1 1 1
  spline S221 degree 2 poles (22.2543, 7.2735) (22.3389, 7.0147) (22.604, 6.9197) knots 0 0 0 1 1 1
  spline S222 degree 2 poles (22.604, 6.9197) (23.0075, 6.7757) (23.4808, 6.9305) knots 0 0 0 1 1 1
  line L134 (23.4808, 6.9305) -> (24.1057, 7.1349)
  line L135 (25.132, -1.2605) -> (24.4746, -1.2619)
  spline S223 degree 2 poles (24.4746, -1.2619) (23.8869, -1.2631) (22.8131, -0.588) (22.8117, 0.0428) knots 0 0 0 1 2 2 2
  spline S224 degree 2 poles (22.8117, 0.0428) (22.811, 0.408) (23.1287, 0.9101) (23.9877, 1.3601) (24.4691, 1.3611) knots 0 0 0 1 2 3 3 3
  line L136 (24.4691, 1.3611) -> (25.1265, 1.3625)
  spline S225 degree 2 poles (25.1265, 1.3625) (25.7109, 1.3637) (26.7881, 0.692) (26.7894, 0.0611) knots 0 0 0 1 2 2 2
  spline S226 degree 2 poles (26.7894, 0.0611) (26.7901, -0.3008) (26.4758, -0.8028) (25.6168, -1.2595) (25.132, -1.2605) knots 0 0 0 1 2 3 3 3
  spline S227 degree 2 poles (25.1308, -0.6595) (25.6222, -0.6585) (25.9868, -0.3855) knots 0 0 0 1 1 1
  spline S228 degree 2 poles (25.9868, -0.3855) (26.189, -0.229) (26.1884, 0.0532) knots 0 0 0 1 1 1
  spline S229 degree 2 poles (26.1884, 0.0532) (26.1878, 0.3288) (25.965, 0.501) knots 0 0 0 1 1 1
  spline S230 degree 2 poles (25.965, 0.501) (25.6258, 0.7626) (25.1278, 0.7615) knots 0 0 0 1 1 1
  line L137 (25.1278, 0.7615) -> (24.4704, 0.7602)
  spline S231 degree 2 poles (24.4704, 0.7602) (23.9756, 0.7591) (23.6143, 0.4828) knots 0 0 0 1 1 1
  spline S232 degree 2 poles (23.6143, 0.4828) (23.4121, 0.3296) (23.4127, 0.0441) knots 0 0 0 1 1 1
  spline S233 degree 2 poles (23.4127, 0.0441) (23.4133, -0.2282) (23.6361, -0.4004) knots 0 0 0 1 1 1
  spline S234 degree 2 poles (23.6361, -0.4004) (23.9753, -0.662) (24.4733, -0.6609) knots 0 0 0 1 1 1
  line L138 (24.4733, -0.6609) -> (25.1308, -0.6595)
  line L139 (26.4213, -4.4368) -> (23.1703, -3.9291)
  line L140 (23.1703, -3.9291) -> (23.0765, -4.5294)
  spline S235 degree 2 poles (23.0765, -4.5294) (23.0417, -4.7525) (22.849, -4.9106) (22.7145, -4.8896) knots 0 0 0 1 2 2 2
  spline S236 degree 2 poles (22.7145, -4.8896) (22.58, -4.8686) (22.4479, -4.6598) (22.4828, -4.4367) knots 0 0 0 1 2 2 2
  line L141 (22.4828, -4.4367) -> (22.763, -2.6423)
  spline S237 degree 2 poles (22.763, -2.6423) (22.7978, -2.4192) (22.9905, -2.2611) (23.125, -2.2821) knots 0 0 0 1 2 2 2
  spline S238 degree 2 poles (23.125, -2.2821) (23.2595, -2.3031) (23.3916, -2.5119) (23.3568, -2.735) knots 0 0 0 1 2 2 2
  line L142 (23.3568, -2.735) -> (23.263, -3.3353)
  line L143 (23.263, -3.3353) -> (25.7398, -3.7221)
  line L144 (25.7398, -3.7221) -> (25.685, -3.1691)
  spline S239 degree 2 poles (25.685, -3.1691) (25.6689, -3.0356) (25.6786, -2.9732) knots 0 0 0 1 1 1
  spline S240 degree 2 poles (25.6786, -2.9732) (25.6966, -2.8584) (25.9026, -2.7226) (26.0338, -2.7431) knots 0 0 0 1 2 2 2
  spline S241 degree 2 poles (26.0338, -2.7431) (26.1519, -2.7615) (26.2675, -2.9039) (26.2897, -3.1056) knots 0 0 0 1 2 2 2
  line L145 (26.2897, -3.1056) -> (26.4213, -4.4368)
  line L146 (25.4026, -8.5134) -> (22.271, -7.5037)
  line L147 (22.271, -7.5037) -> (22.0845, -8.082)
  spline S242 degree 2 poles (22.0845, -8.082) (22.0152, -8.2968) (21.8001, -8.4229) (21.6706, -8.3811) knots 0 0 0 1 2 2 2
  spline S243 degree 2 poles (21.6706, -8.3811) (21.541, -8.3393) (21.4432, -8.1124) (21.5125, -7.8975) knots 0 0 0 1 2 2 2
  line L148 (21.5125, -7.8975) -> (22.0699, -6.169)
  spline S244 degree 2 poles (22.0699, -6.169) (22.1392, -5.9541) (22.3542, -5.8281) (22.4838, -5.8699) knots 0 0 0 1 2 2 2
  spline S245 degree 2 poles (22.4838, -5.8699) (22.6133, -5.9116) (22.7111, -6.1385) (22.6418, -6.3534) knots 0 0 0 1 2 2 2
  line L149 (22.6418, -6.3534) -> (22.4554, -6.9317)
  line L150 (22.4554, -6.9317) -> (24.8412, -7.701)
  line L151 (24.8412, -7.701) -> (24.8736, -7.1463)
  spline S246 degree 2 poles (24.8736, -7.1463) (24.8785, -7.0118) (24.8979, -6.9518) knots 0 0 0 1 1 1
  spline S247 degree 2 poles (24.8979, -6.9518) (24.9336, -6.8412) (25.1583, -6.7392) (25.2847, -6.78) knots 0 0 0 1 2 2 2
  spline S248 degree 2 poles (25.2847, -6.78) (25.3985, -6.8166) (25.4903, -6.9753) (25.4808, -7.1781) knots 0 0 0 1 2 2 2
  line L152 (25.4808, -7.1781) -> (25.4026, -8.5134)
  line L153 (21.8234, -12.5278) -> (21.2369, -12.2307)
  spline S249 degree 2 poles (21.2369, -12.2307) (20.7127, -11.9651) (20.0621, -10.8763) (20.3472, -10.3135) knots 0 0 0 1 2 2 2
  spline S250 degree 2 poles (20.3472, -10.3135) (20.5123, -9.9877) (21.0232, -9.6845) (21.9929, -9.6733) (22.4223, -9.8909) knots 0 0 0 1 2 3 3 3
  line L154 (22.4223, -9.8909) -> (23.0088, -10.1879)
  spline S251 degree 2 poles (23.0088, -10.1879) (23.5301, -10.452) (24.1851, -11.5395) (23.9, -12.1022) knots 0 0 0 1 2 2 2
  spline S252 degree 2 poles (23.9, -12.1022) (23.7365, -12.4251) (23.2285, -12.7297) (22.2558, -12.7469) (21.8234, -12.5278) knots 0 0 0 1 2 3 3 3
  spline S253 degree 2 poles (22.095, -11.9917) (22.5333, -12.2138) (22.9822, -12.136) knots 0 0 0 1 1 1
  spline S254 degree 2 poles (22.9822, -12.136) (23.2334, -12.0883) (23.3609, -11.8365) knots 0 0 0 1 1 1
  spline S255 degree 2 poles (23.3609, -11.8365) (23.4855, -11.5907) (23.365, -11.3362) knots 0 0 0 1 1 1
  spline S256 degree 2 poles (23.365, -11.3362) (23.1815, -10.9491) (22.7372, -10.724) knots 0 0 0 1 1 1
  line L155 (22.7372, -10.724) -> (22.1507, -10.4269)
  spline S257 degree 2 poles (22.1507, -10.4269) (21.7094, -10.2034) (21.262, -10.2857) knots 0 0 0 1 1 1
  spline S258 degree 2 poles (21.262, -10.2857) (21.0123, -10.3304) (20.8833, -10.5851) knots 0 0 0 1 1 1
  spline S259 degree 2 poles (20.8833, -10.5851) (20.7603, -10.828) (20.8807, -11.0825) knots 0 0 0 1 1 1
  spline S260 degree 2 poles (20.8807, -11.0825) (21.0643, -11.4696) (21.5085, -11.6946) knots 0 0 0 1 1 1
  line L156 (21.5085, -11.6946) -> (22.095, -11.9917)
  line L157 (19.5961, -15.786) -> (19.0633, -15.4009)
  spline S261 degree 2 poles (19.0633, -15.4009) (18.5871, -15.0566) (18.1147, -13.8794) (18.4843, -13.3681) knots 0 0 0 1 2 2 2
  spline S262 degree 2 poles (18.4843, -13.3681) (18.6983, -13.0721) (19.2503, -12.8526) (20.2098, -12.9931) (20.6, -13.2751) knots 0 0 0 1 2 3 3 3
  line L158 (20.6, -13.2751) -> (21.1328, -13.6603)
  spline S263 degree 2 poles (21.1328, -13.6603) (21.6064, -14.0026) (22.0833, -15.1791) (21.7138, -15.6903) knots 0 0 0 1 2 2 2
  spline S264 degree 2 poles (21.7138, -15.6903) (21.5017, -15.9836) (20.9524, -16.2052) (19.989, -16.07) (19.5961, -15.786) knots 0 0 0 1 2 3 3 3
  spline S265 degree 2 poles (19.9482, -15.299) (20.3464, -15.5869) (20.8019, -15.5802) knots 0 0 0 1 1 1
  spline S266 degree 2 poles (20.8019, -15.5802) (21.0575, -15.5724) (21.2228, -15.3437) knots 0 0 0 1 1 1
  spline S267 degree 2 poles (21.2228, -15.3437) (21.3843, -15.1203) (21.3051, -14.8501) knots 0 0 0 1 1 1
  spline S268 degree 2 poles (21.3051, -14.8501) (21.1843, -14.4391) (20.7807, -14.1473) knots 0 0 0 1 1 1
  line L159 (20.7807, -14.1473) -> (20.2479, -13.7622)
  spline S269 degree 2 poles (20.2479, -13.7622) (19.847, -13.4723) (19.3923, -13.4837) knots 0 0 0 1 1 1
  spline S270 degree 2 poles (19.3923, -13.4837) (19.1386, -13.4888) (18.9714, -13.7202) knots 0 0 0 1 1 1
  spline S271 degree 2 poles (18.9714, -13.7202) (18.8119, -13.9408) (18.891, -14.2111) knots 0 0 0 1 1 1
  spline S272 degree 2 poles (18.891, -14.2111) (19.0118, -14.6221) (19.4154, -14.9138) knots 0 0 0 1 1 1
  line L160 (19.4154, -14.9138) -> (19.9482, -15.299)
  line L161 (18.7732, -19.1137) -> (16.4408, -16.7929)
  line L162 (16.4408, -16.7929) -> (16.0122, -17.2236)
  spline S273 degree 2 poles (16.0122, -17.2236) (15.853, -17.3836) (15.6042, -17.3983) (15.5077, -17.3023) knots 0 0 0 1 2 2 2
  spline S274 degree 2 poles (15.5077, -17.3023) (15.4112, -17.2063) (15.427, -16.9597) (15.5862, -16.7997) knots 0 0 0 1 2 2 2
  line L163 (15.5862, -16.7997) -> (16.8673, -15.5123)
  spline S275 degree 2 poles (16.8673, -15.5123) (17.0265, -15.3522) (17.2754, -15.3375) (17.3719, -15.4335) knots 0 0 0 1 2 2 2
  spline S276 degree 2 poles (17.3719, -15.4335) (17.4684, -15.5296) (17.4525, -15.7761) (17.2933, -15.9362) knots 0 0 0 1 2 2 2
  line L164 (17.2933, -15.9362) -> (16.8647, -16.3669)
  line L165 (16.8647, -16.3669) -> (18.6417, -18.135)
  line L166 (18.6417, -18.135) -> (18.9222, -17.6554)
  spline S277 degree 2 poles (18.9222, -17.6554) (18.9877, -17.5378) (19.0322, -17.4931) knots 0 0 0 1 1 1
  spline S278 degree 2 poles (19.0322, -17.4931) (19.1141, -17.4107) (19.3607, -17.4219) (19.4548, -17.5156) knots 0 0 0 1 2 2 2
  spline S279 degree 2 poles (19.4548, -17.5156) (19.5395, -17.5999) (19.5494, -17.783) (19.4489, -17.9593) knots 0 0 0 1 2 2 2
  line L167 (19.4489, -17.9593) -> (18.7732, -19.1137)
  line L168 (13.7621, -21.0668) -> (13.3743, -20.536)
  spline S280 degree 2 poles (13.3743, -20.536) (13.0277, -20.0614) (12.942, -18.7959) (13.4515, -18.4238) knots 0 0 0 1 2 2 2
  spline S281 degree 2 poles (13.4515, -18.4238) (13.7464, -18.2083) (14.3393, -18.17) (15.2085, -18.6) (15.4924, -18.9888) knots 0 0 0 1 2 3 3 3
  line L169 (15.4924, -18.9888) -> (15.8802, -19.5197)
  spline S282 degree 2 poles (15.8802, -19.5197) (16.2249, -19.9915) (16.3152, -21.2578) (15.8057, -21.6299) knots 0 0 0 1 2 2 2
  spline S283 degree 2 poles (15.8057, -21.6299) (15.5135, -21.8434) (14.9226, -21.8844) (14.048, -21.4583) (13.7621, -21.0668) knots 0 0 0 1 2 3 3 3
  spline S284 degree 2 poles (14.2474, -20.7124) (14.5372, -21.1092) (14.9725, -21.2435) knots 0 0 0 1 1 1
  spline S285 degree 2 poles (14.9725, -21.2435) (15.218, -21.315) (15.4459, -21.1485) knots 0 0 0 1 1 1
  spline S286 degree 2 poles (15.4459, -21.1485) (15.6684, -20.986) (15.6766, -20.7045) knots 0 0 0 1 1 1
  spline S287 degree 2 poles (15.6766, -20.7045) (15.6887, -20.2763) (15.3949, -19.8741) knots 0 0 0 1 1 1
  line L170 (15.3949, -19.8741) -> (15.0071, -19.3433)
  spline S288 degree 2 poles (15.0071, -19.3433) (14.7153, -18.9438) (14.2793, -18.8141) knots 0 0 0 1 1 1
  spline S289 degree 2 poles (14.2793, -18.8141) (14.0365, -18.7406) (13.8059, -18.9091) knots 0 0 0 1 1 1
  spline S290 degree 2 poles (13.8059, -18.9091) (13.5861, -19.0696) (13.5779, -19.3511) knots 0 0 0 1 1 1
  spline S291 degree 2 poles (13.5779, -19.3511) (13.5658, -19.7793) (13.8596, -20.1815) knots 0 0 0 1 1 1
  line L171 (13.8596, -20.1815) -> (14.2474, -20.7124)
  line L172 (11.9516, -23.9777) -> (10.4501, -21.0499)
  line L173 (10.4501, -21.0499) -> (9.9094, -21.3271)
  spline S292 degree 2 poles (9.9094, -21.3271) (9.7085, -21.4302) (9.4673, -21.3673) (9.4052, -21.2462) knots 0 0 0 1 2 2 2
  spline S293 degree 2 poles (9.4052, -21.2462) (9.3431, -21.125) (9.4343, -20.8954) (9.6352, -20.7924) knots 0 0 0 1 2 2 2
  line L174 (9.6352, -20.7924) -> (11.2512, -19.9636)
  spline S294 degree 2 poles (11.2512, -19.9636) (11.4521, -19.8606) (11.6933, -19.9234) (11.7555, -20.0446) knots 0 0 0 1 2 2 2
  spline S295 degree 2 poles (11.7555, -20.0446) (11.8176, -20.1657) (11.7264, -20.3953) (11.5255, -20.4983) knots 0 0 0 1 2 2 2
  line L175 (11.5255, -20.4983) -> (10.9848, -20.7756)
  line L176 (10.9848, -20.7756) -> (12.1288, -23.0062)
  line L177 (12.1288, -23.0062) -> (12.5437, -22.6367)
  spline S296 degree 2 poles (12.5437, -22.6367) (12.6423, -22.5451) (12.6984, -22.5163) knots 0 0 0 1 1 1
  spline S297 degree 2 poles (12.6984, -22.5163) (12.8018, -22.4632) (13.0329, -22.55) (13.0935, -22.6682) knots 0 0 0 1 2 2 2
  spline S298 degree 2 poles (13.0935, -22.6682) (13.148, -22.7745) (13.1008, -22.9517) (12.9508, -23.0884) knots 0 0 0 1 2 2 2
  line L178 (12.9508, -23.0884) -> (11.9516, -23.9777)
  dimension "d7" = 1.905
  constraints: 1 centre point, 1 coincident, 1 other
  measures "d7" radial gap between concentric circles of A2 A3
extrude "Extrusion1" cut sketch "Sketch2" along normal blind 25.4 contours A3 S223 S224 | A3 S224 L136 S225 S226 L135 S223 | L141 S237 S238 L142 L143 L144 S239 S240 S241 L145 L139 L140 S235 S236 | L148 S244 S245 L149 L150 L151 S246 S247 S248 L152 L146 L147 S242 S243 | L163 S275 S276 L164 L165 L166 S277 S278 S279 L167 L161 L162 S273 S274 | L174 S294 S295 L175 L176 L177 S296 S297 S298 L178 L172 L173 S292 S293 | L6 S14 S15 L7 L8 L9 S16 S17 S18 L10 L4 L5 S12 S13 | L13 S21 S22 L14 L15 L16 S23 S24 S25 L17 L11 L12 S19 S20 | L32 S64 S65 L33 L34 L35 S66 S67 S68 L36 L30 L31 S62 S63 | L39 S71 S72 L40 L41 L42 S73 S74 S75 L43 L37 L38 S69 S70 | L50 S90 S91 L51 L52 L53 S92 S93 S94 L54 L48 L49 S88 S89 | L57 S97 S98 L58 L59 L60 S99 S100 S101 L61 L55 L56 S95 S96 | L68 S116 S117 L69 L70 L71 S118 S119 S120 L72 L66 L67 S114 S115 | L75 S123 S124 L76 L77 L78 S125 S126 S127 L79 L73 L74 S121 S122 | L82 S130 S131 L83 L84 L85 S132 S133 S134 L86 L80 L81 S128 S129 | L89 S137 S138 L90 L91 L92 S139 S140 S141 L93 L87 L88 S135 S136 | L100 S156 S157 L101 L102 L103 S158 S159 S160 L104 L98 L99 S154 S155 | L107 S163 S164 L108 L109 L110 S165 S166 S167 L111 L105 L106 S161 S162 | L122 S194 S195 L123 L124 L125 S196 S197 S198 L126 L120 L121 S192 S193 | S211 S212 A3 | A3 S212 L132 S213 S214 L131 S211 | S199 S200 A3 | A3 S200 L128 S201 S202 L127 S199 | S250 L154 S251 S252 L153 S249 A3 | A3 S249 S250 | S262 L158 S263 S264 L157 S261 A3 | A3 S261 S262 | S180 S181 A3 | A3 S181 L117 S182 S183 L116 S180 | S168 S169 A3 | A3 S169 L113 S170 S171 L112 S168 | S281 L169 S282 S283 L168 S280 A3 | A3 S280 S281 | S1 L1 S2 S3 L0 S0 A3 | A3 S0 S1 | S142 S143 A3 | A3 S143 L95 S144 S145 L94 S142 | S27 L19 S28 S29 L18 S26 A3 | A3 S26 S27 | S39 L23 S40 S41 L22 S38 A3 | A3 S38 S39 | S102 S103 A3 | A3 S103 L63 S104 S105 L62 S102 | S51 L27 S52 S53 L26 S50 A3 | A3 S50 S51 | S76 S77 A3 | A3 S77 L45 S78 S79 L44 S76 keep common part
body "Solid1"
